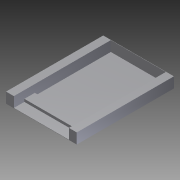
# Autodesk Inventor part: Concept
Saved by Autodesk Inventor 2012 (Build 160160000, 160)
## iProperties
Created: 2011-09-11
Part Number: Concept
Material: Default
Document SubType Name: Modeling
Designer: Ian Walters
Density: 1 g/cm^3
Author: Ian Walters
Autodesk Inventor part; units mm, degrees
ref_plane "YZ Plane" through (0, 0, 0) normal (1, 0, 0) x (0, 1, 0)
ref_plane "XZ Plane" through (0, 0, 0) normal (0, 1, 0) x (-1, 0, 0)
ref_plane "XY Plane" through (0, 0, 0) normal (0, 0, 1) x (1, 0, 0)
sketch "Sketch1" plane through (0, 0, 0) normal (0, 0, 1) x (1, 0, 0)
  line L0 (-266.7, 101.6) -> (-342.9, 101.6)
  line L1 (-342.9, 101.6) -> (-342.9, 0)
  line L2 (-342.9, 0) -> (342.9, 0)
  line L3 (342.9, 0) -> (342.9, 101.6)
  line L4 (342.9, 101.6) -> (266.7, 101.6)
  line L5 (266.7, 101.6) -> (266.7, 2.54)
  line L6 (266.7, 2.54) -> (-266.7, 2.54)
  line L7 (-266.7, 2.54) -> (-266.7, 101.6)
  point P0 (0, 0)
  point P1 (0, 0)
  point P2 (0, 2.54)
  dimension "d0" = 685.8
  dimension "d1" = 101.6
  dimension "d2" = 76.2
  dimension "d3" = 2.54
  constraints: 16 end point, 5 parallel, 2 collinear, 2 midpoint, 1 coincident, 1 horizontal, 1 perpendicular, 1 vertical alignment
  measures "d0" distance of L1.end L2.end
  measures "d1" distance of L0.end L1.end
  measures "d2" distance of L0.start L0.end
  measures "d3" distance between parallel lines of L2 L6
extrude "Extrusion1" add sketch "Sketch1" along normal mid plane 939.8
sketch "Sketch2" plane through (0, 0, -469.9) normal (0, 0, -1) x (-1, 0, 0)
  line L0 (-342.9, 0) -> (-342.9, 101.6) projected
  line L1 (342.9, 0) -> (-342.9, 0) projected
  line L2 (-342.9, 101.6) -> (342.9, 101.6)
  line L3 (342.9, 101.6) -> (342.9, 0)
  line L4 (342.9, 0) -> (-342.9, 0)
  line L5 (-342.9, 0) -> (-342.9, 101.6)
  point P0 (0, 0)
  constraints: 8 end point, 2 parallel, 1 horizontal, 1 perpendicular
extrude "Extrusion2" add sketch "Sketch2" along normal blind 2.54
sketch "Sketch3" plane through (-266.7, 2.54, 469.9) normal (0, 1, 0) x (1, 0, 0)
  line L0 (0, 0) -> (533.4, 0) projected
  line L1 (533.4, 939.8) -> (533.4, 0) projected
  line L2 (0, 939.8) -> (0, 0) projected
  line L3 (0, 101.6) -> (533.4, 101.6)
  line L4 (533.4, 101.6) -> (533.4, 203.2)
  line L5 (533.4, 203.2) -> (0, 203.2)
  line L6 (0, 203.2) -> (0, 101.6)
  point P0 (266.7, 469.9)
  dimension "d8" = 101.6
  dimension "d9" = 101.6
  constraints: 8 end point, 2 parallel, 2 point on line, 1 horizontal, 1 perpendicular
  measures "d8" distance of L5.end L3.start
  measures "d9" distance between parallel lines of L0 L3
extrude "Extrusion3" add sketch "Sketch3" along normal blind 25.4 contours L2 L5 L1 L3
sketch "Sketch4" plane through (-342.9, 0, 469.9) normal (0, -1, 0) x (1, 0, 0)
  line L0 (685.8, 0) -> (0, 0) projected
  line L1 (0, -942.34) -> (0, 0) projected
  line L2 (0, -942.34) -> (685.8, -942.34) projected
  line L3 (76.2, -939.8) -> (76.2, -203.2) projected
  line L4 (342.9, -469.9) -> (342.9, 0) construction
  line L5 (12.7, -929.64) -> (63.5, -929.64)
  line L6 (63.5, -929.64) -> (63.5, -12.7)
  line L7 (63.5, -12.7) -> (12.7, -12.7)
  line L8 (12.7, -12.7) -> (12.7, -929.64)
  line L9 (673.1, -929.64) -> (622.3, -929.64)
  line L10 (622.3, -929.64) -> (622.3, -12.7)
  line L11 (622.3, -12.7) -> (673.1, -12.7)
  line L12 (673.1, -12.7) -> (673.1, -929.64)
  dimension "d12" = 12.7
  dimension "d13" = 12.7
  dimension "d14" = 12.7
  dimension "d15" = 12.7
  constraints: 18 end point, 4 symmetric about line, 2 parallel, 1 horizontal, 1 midpoint, 1 perpendicular
  measures "d12" distance between parallel lines of L1 L8
  measures "d13" distance between parallel lines of L3 L6
  measures "d14" distance between parallel lines of L0 L7
  measures "d15" distance between parallel lines of L5 L2
extrude "Extrusion4" cut sketch "Sketch4" against normal blind 88.9
body "Solid1"
